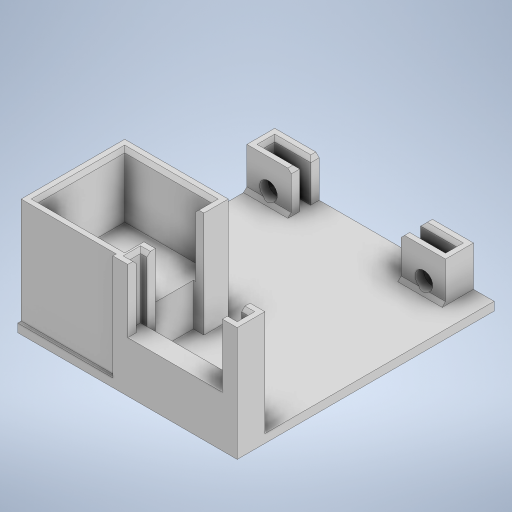
# Autodesk Inventor part: testbench
Saved by Autodesk Inventor 2023 (Build 270158000, 158)
## iProperties
Created: 2023-01-23
Part Number: testbench
Material: Generic
Document SubType Name: Modeling
Designer: karpova
Density: 1 g/cm^3
Appearance: Default
Author: karpova
Autodesk Inventor part; units mm, degrees
ref_plane "YZ Plane" through (0, 0, 0) normal (1, 0, 0) x (0, 1, 0)
ref_plane "XZ Plane" through (0, 0, 0) normal (0, 1, 0) x (-1, 0, 0)
ref_plane "XY Plane" through (0, 0, 0) normal (0, 0, 1) x (1, 0, 0)
sketch "Sketch1" plane through (0, 0, 0) normal (0, 1, 0) x (-1, 0, 0)
  line L0 (31.9073, 34.2364) -> (-15.0927, 34.2364)
  line L1 (-15.0927, 34.2364) -> (-15.0927, -25.7636)
  line L2 (-15.0927, -25.7636) -> (31.9073, -25.7636)
  line L3 (31.9073, -25.7636) -> (31.9073, 34.2364)
  point P0 (0, 0)
  dimension "d0" = 47
  dimension "d60" = 60
  constraints: 8 end point, 2 parallel, 1 horizontal, 1 perpendicular
  measures "d0" distance of L1.end L2.end
  measures "d60" distance of L2.end L0.start
extrude "Extrusion1" add sketch "Sketch1" along normal blind 2
sketch "Sketch2" plane through (0, 2, 0) normal (0, 1, 0) x (1, 0, 0)
  line L0 (13.0927, 21.1636) -> (-29.9073, 21.1636)
  line L1 (-29.9073, 21.1636) -> (-29.9073, 23.7636)
  line L2 (-29.9073, 23.7636) -> (13.0927, 23.7636)
  line L3 (13.0927, 23.7636) -> (13.0927, 21.1636)
  line L4 (15.0927, 25.7636) -> (-31.9073, 25.7636)
  line L5 (-31.9073, 25.7636) -> (-31.9073, 19.1636)
  line L6 (-31.9073, 19.1636) -> (15.0927, 19.1636)
  line L7 (15.0927, 19.1636) -> (15.0927, 25.7636)
  line L8 (15.0927, -34.2364) -> (15.0927, 25.7636) projected
  line L9 (15.0927, 25.7636) -> (-31.9073, 25.7636) projected
  point P0 (0, 0)
  dimension "d3" = 43
  dimension "d4" = 2.6
  dimension "d5" = 2
  dimension "d6" = 0
  dimension "d7" = 0
  constraints: 16 end point, 4 parallel, 2 perpendicular, 1 horizontal, 3 other
  measures "d3" distance of L1.end L2.end
  measures "d4" distance between parallel lines of L2 L0
  measures "d5" distance between parallel lines of L4 L2
  measures "d6" distance between parallel lines of L8 L7
  measures "d7" distance between parallel lines of L9 L4
extrude "Extrusion2" add sketch "Sketch2" along normal blind 9.5
sketch "Sketch3" plane through (15.0927, 0, -25.7636) normal (0, 0, -1) x (-1, 0, 0)
  circle A0 centre (5.1104, 4.5356) radius 1.6 construction
  circle A1 centre (41.8896, 4.5356) radius 1.6 construction
  line L0 (0, 0) -> (47, 0) construction
  line L1 (23.5, 0) -> (23.5, 11.5) construction
  line L2 (0, 11.5) -> (47, 11.5) construction
  line L3 (2, 2) -> (2, 11.5) construction
  line L4 (2, 2) -> (45, 2) construction
  line L5 (45, 2) -> (45, 11.5) construction
  line L6 (2.5, 2) -> (44.5, 2) construction
  line L7 (44.5, 2) -> (44.5, 47) construction
  line L8 (44.5, 47) -> (2.5, 47) construction
  line L9 (2.5, 47) -> (2.5, 2) construction
  line L10 (2.5, 24.5) -> (44.5, 24.5) construction
  circle A2 centre (5.1104, 4.5356) radius 2.1
  circle A3 centre (41.8896, 4.5356) radius 2.1
  point P0 (15.0927, 0)
  dimension "d10" = 36.7792
  dimension "d11" = 42
  dimension "d12" = 45
  dimension "d13" = 19.9644
  dimension "d14" = 3.2
  dimension "d15" = 0.5
  constraints: 12 end point, 4 centre point, 4 midpoint, 2 coincident, 2 equal radius, 2 parallel, 1 collinear, 1 horizontal, 1 perpendicular, 1 symmetric about line, 1 other
  measures "d10" distance of A1.centre A0.centre
  measures "d11" distance of L7.end L8.end
  measures "d12" distance of L8.end L6.start
  measures "d13" distance from line of A0.centre L10
  measures "d14" diameter of A0
  measures "d15" radial gap between concentric circles of A2 A0
extrude "Extrusion3" cut sketch "Sketch3" against normal blind 15
chamfer "Chamfer1" distance 0.8 angle 45 4 edges at (-8.4073, 11.5, -21.1636) (-8.4073, 11.5, -23.7636) (13.0927, 11.5, -22.4636) (-29.9073, 11.5, -22.4636)
sketch "Sketch4" plane through (-31.9073, 11.5, -19.1636) normal (0, 0, 1) x (1, 0, 0)
  line L0 (0, 0) -> (47, 0) projected
  line L1 (47, -9.5) -> (0, -9.5) projected
  line L2 (10.5, 0) -> (36.5, 0)
  line L3 (36.5, 0) -> (36.5, -9.5)
  line L4 (36.5, -9.5) -> (10.5, -9.5)
  line L5 (10.5, -9.5) -> (10.5, 0)
  line L6 (47, -9.5) -> (47, 0) construction
  line L7 (45.8, 0) -> (1.2, 0) construction
  line L8 (23.5, 0) -> (23.5, -9.5) construction
  point P0 (31.9073, -11.5)
  point P1 (41.3145, -9.5)
  point P2 (5.6855, -9.5)
  point P3 (10.5, -9.5)
  point P4 (36.5, 0)
  dimension "d21" = 10.5
  constraints: 10 end point, 2 midpoint, 2 parallel, 2 point on line, 1 horizontal, 1 perpendicular, 1 other
  measures "d21" distance between parallel lines of L6 L3
extrude "Extrusion4" cut sketch "Sketch4" against normal through all
chamfer "Chamfer2" distance 0.8 angle 45 6 edges at (-21.4073, 11.5, -19.7636) (4.5927, 11.5, -19.7636) (9.8427, 2, -19.1636) (-26.6573, 2, -19.1636) (-21.4073, 11.5, -25.1636) (4.5927, 11.5, -25.1636)
sketch "Sketch5" plane through (0, 2, 0) normal (0, 1, 0) x (1, 0, 0)
  line L0 (-29.9073, -11.7364) -> (-9.4073, -11.7364)
  line L1 (-9.4073, -11.7364) -> (-9.4073, -32.2364)
  line L2 (-9.4073, -32.2364) -> (-29.9073, -32.2364)
  line L3 (-29.9073, -32.2364) -> (-29.9073, -11.7364)
  line L4 (-7.4073, -9.7364) -> (-31.9073, -9.7364)
  line L5 (-31.9073, -9.7364) -> (-31.9073, -34.2364)
  line L6 (-31.9073, -34.2364) -> (-7.4073, -34.2364)
  line L7 (-7.4073, -34.2364) -> (-7.4073, -9.7364)
  line L8 (-31.9073, 19.1636) -> (-31.9073, -34.2364) projected
  line L9 (-31.9073, -34.2364) -> (15.0927, -34.2364) projected
  point P0 (0, 0)
  point P1 (-31.9073, 16.9636)
  point P2 (-31.9073, 25.7636)
  dimension "d27" = 20.5
  dimension "d28" = 2
  dimension "d29" = 0
  dimension "d30" = 0
  constraints: 16 end point, 4 parallel, 3 perpendicular, 1 horizontal, 3 other
  measures "d27" distance of L0.end L1.end
  measures "d28" distance between parallel lines of L4 L0
  measures "d29" distance between parallel lines of L8 L5
  measures "d30" distance between parallel lines of L9 L6
extrude "Extrusion5" add sketch "Sketch5" along normal blind 25
sketch "Sketch6" plane through (0, 2, 0) normal (0, 1, 0) x (1, 0, 0)
  line L0 (-29.9073, -11.7364) -> (-29.9073, -32.2364) projected
  line L1 (-29.9073, -32.2364) -> (-9.4073, -32.2364) projected
  line L2 (-9.4073, -32.2364) -> (-9.4073, -11.7364) projected
  line L3 (-9.4073, -11.7364) -> (-29.9073, -11.7364) projected
  point P0 (0, 0)
extrude "Extrusion6" add sketch "Sketch6" along normal blind 10
sketch "Sketch7" plane through (-7.4073, 2, 34.2364) normal (1, 0, 0) x (0, 0, -1)
  line L0 (22.5, 10) -> (2, 10) projected
  line L1 (2, 25) -> (22.5, 25) projected
  line L2 (5.75, 25) -> (18.75, 25)
  line L3 (18.75, 25) -> (18.75, 0)
  line L4 (18.75, 0) -> (5.75, 0)
  line L5 (5.75, 0) -> (5.75, 25)
  line L6 (24.5, 0) -> (0, 0) construction
  line L7 (12.25, 0) -> (12.25, 25) construction
  line L8 (0, 0) -> (52.6, 0) construction
  point P0 (34.2364, -2)
  point P1 (51.2, 0)
  dimension "d35" = 13
  constraints: 10 end point, 2 midpoint, 2 parallel, 1 collinear, 1 horizontal, 1 perpendicular, 1 point on line, 1 vertical, 1 other
  measures "d35" distance between parallel lines of L3 L5
extrude "Extrusion7" cut sketch "Sketch7" against normal blind 2.5
sketch "Sketch8" plane through (0, 2, 0) normal (0, 1, 0) x (1, 0, 0)
  line L0 (-7.4073, -30.4864) -> (17.9927, -30.4864)
  line L1 (17.9927, -30.4864) -> (17.9927, -33.0264)
  line L2 (17.9927, -33.0264) -> (-7.4073, -33.0264)
  line L3 (-7.4073, -33.0264) -> (-7.4073, -30.4864)
  line L4 (19.9927, -28.4864) -> (-9.4073, -28.4864)
  line L5 (-9.4073, -28.4864) -> (-9.4073, -35.0264)
  line L6 (-9.4073, -35.0264) -> (19.9927, -35.0264)
  line L7 (19.9927, -35.0264) -> (19.9927, -28.4864)
  line L8 (-7.4073, -34.2364) -> (-7.4073, -9.7364) projected
  line L9 (-7.4073, -34.2364) -> (15.0927, -34.2364) projected
  line L10 (-7.4073, -28.4864) -> (-9.4073, -28.4864) projected
  point P0 (0, 0)
  dimension "d41" = 25.4
  dimension "d42" = 2.54
  dimension "d43" = 2
  constraints: 16 end point, 4 parallel, 2 collinear, 2 perpendicular, 1 horizontal, 3 other
  measures "d41" distance of L1.end L2.end
  measures "d42" distance between parallel lines of L0 L2
  measures "d43" distance between parallel lines of L5 L3
extrude "Extrusion8" add sketch "Sketch8" along normal up to surface (25 mm away)
sketch "Sketch9" plane through (15.0927, 0, 34.2364) normal (1, 0, 0) x (0, 0, -1)
  line L0 (0, 2) -> (-0.79, 2) projected
  line L1 (-0.79, 2) -> (60, 2)
  line L2 (60, 2) -> (60, 0)
  line L3 (60, 0) -> (-0.79, 0)
  line L4 (-0.79, 0) -> (-0.79, 2)
  point P0 (34.2364, 0)
  constraints: 8 end point, 2 parallel, 1 horizontal, 1 perpendicular
extrude "Extrusion9" add sketch "Sketch9" along normal up to surface (4.9 mm away)
sketch "Sketch11" plane through (-9.4073, 12, 28.4864) normal (0, 0, -1) x (-1, 0, 0)
  line L0 (-27.4, -10) -> (-27.4, 15) projected
  line L1 (-2, -10) -> (-2, 15) projected
  line L2 (-2, -10) -> (-27.4, -10) construction
  line L3 (-2, 15) -> (0, 15) construction
  line L4 (-25.9, 15) -> (-3.5, 15)
  line L5 (-3.5, 15) -> (-3.5, -10)
  line L6 (-3.5, -10) -> (-25.9, -10)
  line L7 (-25.9, -10) -> (-25.9, 15)
  point P0 (-9.4073, -12)
  point P1 (-29.4, 15)
  dimension "d50" = 1.5
  dimension "d63" = 1.5
  constraints: 8 end point, 2 collinear, 2 parallel, 1 horizontal, 1 perpendicular
  measures "d50" distance between parallel lines of L7 L0
  measures "d63" distance between parallel lines of L1 L5
extrude "Extrusion11" cut sketch "Sketch11" against normal up to surface (2 mm away)
sketch "Sketch12" plane through (-31.9073, 0, 35.0264) normal (0, 0, 1) x (1, 0, 0)
  line L0 (26, 27) -> (48.4, 27)
  line L1 (48.4, 27) -> (48.4, 2)
  line L2 (48.4, 2) -> (26, 2)
  line L3 (26, 2) -> (26, 27)
  line L4 (0, 2) -> (22.5, 2) projected
  line L5 (26, 2) -> (26, 27) projected
  line L6 (48.4, 27) -> (48.4, 2) projected
  line L7 (51.9, 27) -> (22.5, 27) projected
  line L8 (22.5, 2) -> (47, 2) projected
  point P0 (31.9073, 0)
  constraints: 8 end point, 4 collinear, 2 parallel, 1 horizontal, 1 perpendicular
extrude "Extrusion12" cut sketch "Sketch12" against normal up to surface (2 mm away)
sketch "Sketch13" plane through (0, 2, 0) normal (0, 1, 0) x (1, 0, 0)
  line L0 (-7.4073, -30.4864) -> (17.9927, -30.4864) projected
  line L1 (-7.4073, -30.4864) -> (17.9927, -30.4864)
  line L2 (17.9927, -30.4864) -> (17.9927, -35.0264)
  line L3 (17.9927, -35.0264) -> (-7.4073, -35.0264)
  line L4 (-7.4073, -35.0264) -> (-7.4073, -30.4864)
  line L5 (17.9927, -33.0264) -> (17.9927, -30.4864) projected
  line L6 (16.4927, -35.0264) -> (15.0927, -35.0264) projected
  point P0 (0, 0)
  point P1 (-1.9073, -23.0464)
  point P2 (-0.9073, -18.5064)
  constraints: 8 end point, 2 collinear, 2 parallel, 1 horizontal, 1 perpendicular
extrude "Extrusion13" add sketch "Sketch13" along normal blind 10
chamfer "Chamfer4" distance 0.8 angle 45 11 edges at (-9.4073, 27, 30.3614) (-19.6573, 27, 32.2364) (-29.9073, 27, 21.9864) (-19.6573, 27, 11.7364) (-9.4073, 27, 13.6114) (-7.4073, 27, 31.7564) (-6.6573, 27, 33.0264) (-6.6573, 27, 30.4864) (17.2427, 27, 33.0264) (17.2427, 27, 30.4864) (17.9927, 27, 31.7564)
sketch "Sketch14" plane through (-31.9073, 0, 34.2364) normal (0, 0, 1) x (1, 0, 0)
  line L0 (47, 0) -> (47, 2) projected
  line L1 (0, 2.8) -> (0, 11.5) projected
  line L2 (47, 0) -> (0, 0)
  line L3 (0, 0) -> (0, 2)
  line L4 (0, 2) -> (47, 2)
  line L5 (47, 2) -> (47, 0)
  line L6 (22.5, 2) -> (47, 2) projected
  point P0 (31.9073, 0)
  constraints: 8 end point, 2 parallel, 1 collinear, 1 horizontal, 1 perpendicular, 1 point on line
extrude "Extrusion14" add sketch "Sketch14" along normal up to surface (0.79 mm away)
equation "\"d1\" = wallthickness"
equation "\"d4\" = pcbThickness + 2 * clearance"
equation "\"d5\" = wallthickness"
equation "\"d14\" = mountHoleDiameter"
equation "\"d15\" = clearance"
equation "\"d18\" = 0.4 * wallthickness"
equation "\"d21\" = stepperMotorDriverEdgeOffset - clearance"
equation "\"d24\" = 0.4 * wallthickness"
equation "\"d28\" = wallthickness"
equation "\"d36\" = wallthickness + clearance"
equation "\"d43\" = wallthickness"
equation "\"d57\" = 0.4 * wallthickness"
equation "\"wallthickness\" = 2"
equation "\"clearance\" = 0.5"
equation "\"pcbThickness\" = 1.6"
equation "\"mountHoleDiameter\" = 3.2"
equation "\"stepperMotorDriverEdgeOffset\" = 11"
body "Solid1"
